Autodesk Fusion 360 part; units mm, degrees
(part 4 of 4)
sketch "Sketch10" plane through (0, 0, 4.8) normal (0, 0, 1) x (-1, 0, 0)
  circle A0 centre (0, 0) radius 3
  line L0 (57.7941, -61.1213) -> (57.7941, -86.8787)
  arc A1 (55.6728, -89) -> (57.7941, -86.8787) centre (56.7335, -87.9393) ccw
  line L1 (55.6728, -89) -> (53.2941, -89)
  line L2 (53.2941, -89) -> (53.2941, -89.8787)
  arc A2 (51.1728, -92) -> (53.2941, -89.8787) centre (52.2335, -90.9393) ccw
  line L3 (51.1728, -92) -> (18.4155, -92)
  arc A3 (16.2941, -89.8787) -> (18.4155, -92) centre (17.3548, -90.9393) ccw
  line L4 (16.2941, -89.8787) -> (16.2941, -89)
  line L5 (16.2941, -89) -> (13.9155, -89)
  arc A4 (11.7941, -86.8787) -> (13.9155, -89) centre (12.8548, -87.9393) ccw
  line L6 (11.7941, -86.8787) -> (11.7941, -61.1213)
  arc A5 (13.9155, -59) -> (11.7941, -61.1213) centre (12.8548, -60.0607) ccw
  line L7 (13.9155, -59) -> (16.2941, -59)
  line L8 (16.2941, -59) -> (16.2941, -58.1213)
  arc A6 (18.4155, -56) -> (16.2941, -58.1213) centre (17.3548, -57.0607) ccw
  line L9 (18.4155, -56) -> (51.1728, -56)
  arc A7 (53.2941, -58.1213) -> (51.1728, -56) centre (52.2335, -57.0607) ccw
  line L10 (53.2941, -58.1213) -> (53.2941, -59)
  line L11 (53.2941, -59) -> (55.6728, -59)
  arc A8 (57.7941, -61.1213) -> (55.6728, -59) centre (56.7335, -60.0607) ccw
  line L12 (51.1728, 56) -> (18.4155, 56)
  arc A9 (16.2941, 58.1213) -> (18.4155, 56) centre (17.3548, 57.0607) ccw
  line L13 (16.2941, 58.1213) -> (16.2941, 59)
  line L14 (16.2941, 59) -> (13.9155, 59)
  arc A10 (11.7941, 61.1213) -> (13.9155, 59) centre (12.8548, 60.0607) ccw
  line L15 (11.7941, 61.1213) -> (11.7941, 86.8787)
  arc A11 (13.9155, 89) -> (11.7941, 86.8787) centre (12.8548, 87.9393) ccw
  line L16 (13.9155, 89) -> (16.2941, 89)
  line L17 (16.2941, 89) -> (16.2941, 89.8787)
  arc A12 (18.4155, 92) -> (16.2941, 89.8787) centre (17.3548, 90.9393) ccw
  line L18 (18.4155, 92) -> (51.1728, 92)
  arc A13 (53.2941, 89.8787) -> (51.1728, 92) centre (52.2335, 90.9393) ccw
  line L19 (53.2941, 89.8787) -> (53.2941, 89)
  line L20 (53.2941, 89) -> (55.6728, 89)
  arc A14 (57.7941, 86.8787) -> (55.6728, 89) centre (56.7335, 87.9393) ccw
  line L21 (57.7941, 86.8787) -> (57.7941, 61.1213)
  arc A15 (55.6728, 59) -> (57.7941, 61.1213) centre (56.7335, 60.0607) ccw
  line L22 (55.6728, 59) -> (53.2941, 59)
  line L23 (53.2941, 59) -> (53.2941, 58.1213)
  arc A16 (51.1728, 56) -> (53.2941, 58.1213) centre (52.2335, 57.0607) ccw
  arc A17 (65.7941, 74.3) -> (67.2941, 72.8) centre (67.2941, 74.3) ccw
  line L24 (65.7941, 74.3) -> (65.7941, 100.26)
  arc A18 (68.1301, 101.5054) -> (65.7941, 100.26) centre (67.2941, 100.26) ccw
  arc A19 (96.3668, 75.223) -> (68.1301, 101.5054) centre (0, 0) ccw
  arc A20 (95.1844, 72.8) -> (96.3668, 75.223) centre (95.1844, 74.3) ccw
  line L25 (95.1844, 72.8) -> (67.2941, 72.8)
  arc A21 (65.7941, -100.26) -> (68.1301, -101.5054) centre (67.2941, -100.26) ccw
  line L26 (65.7941, -100.26) -> (65.7941, -74.3)
  arc A22 (67.2941, -72.8) -> (65.7941, -74.3) centre (67.2941, -74.3) ccw
  line L27 (67.2941, -72.8) -> (95.1844, -72.8)
  arc A23 (96.3668, -75.223) -> (95.1844, -72.8) centre (95.1844, -74.3) ccw
  arc A24 (68.1301, -101.5054) -> (96.3668, -75.223) centre (0, 0) ccw
  circle A25 centre (64.2941, -62.4) radius 1.5
  circle A26 centre (64.2941, 62.4) radius 1.5
  circle A27 centre (97.2941, -62.4) radius 1.5
  circle A28 centre (97.2941, 62.4) radius 1.5
  circle A29 centre (1.7941, -104.2) radius 6.1
  line L28 (15.4941, 111.4) -> (41.8941, 111.4)
  arc A30 (45.5941, 107.7) -> (41.8941, 111.4) centre (41.8941, 107.7) ccw
  line L29 (45.5941, 107.7) -> (45.5941, 100.7)
  arc A31 (41.8941, 97) -> (45.5941, 100.7) centre (41.8941, 100.7) ccw
  line L30 (41.8941, 97) -> (15.4941, 97)
  arc A32 (11.7941, 100.7) -> (15.4941, 97) centre (15.4941, 100.7) ccw
  line L31 (11.7941, 100.7) -> (11.7941, 107.7)
  arc A33 (15.4941, 111.4) -> (11.7941, 107.7) centre (15.4941, 107.7) ccw
  line L32 (15.4941, -97) -> (41.8941, -97)
  arc A34 (45.5941, -100.7) -> (41.8941, -97) centre (41.8941, -100.7) ccw
  line L33 (45.5941, -100.7) -> (45.5941, -107.7)
  arc A35 (41.8941, -111.4) -> (45.5941, -107.7) centre (41.8941, -107.7) ccw
  line L34 (41.8941, -111.4) -> (15.4941, -111.4)
  arc A36 (11.7941, -107.7) -> (15.4941, -111.4) centre (15.4941, -107.7) ccw
  line L35 (11.7941, -107.7) -> (11.7941, -100.7)
  arc A37 (15.4941, -97) -> (11.7941, -100.7) centre (15.4941, -100.7) ccw
  arc A38 (94.6728, -10) -> (96.7941, -7.8787) centre (95.7335, -8.9393) ccw
  line L36 (94.6728, -10) -> (94.1155, -10)
  arc A39 (91.9941, -7.8787) -> (94.1155, -10) centre (93.0548, -8.9393) ccw
  line L37 (91.9941, -7.8787) -> (91.9941, 7.8787)
  arc A40 (94.1155, 10) -> (91.9941, 7.8787) centre (93.0548, 8.9393) ccw
  line L38 (94.1155, 10) -> (94.6728, 10)
  arc A41 (96.7941, 7.8787) -> (94.6728, 10) centre (95.7335, 8.9393) ccw
  line L39 (96.7941, 7.8787) -> (96.7941, -7.8787)
  circle A42 centre (-94.9024, 87.3758) radius 1.5
  circle A43 centre (123.1209, -38.5) radius 1.5
  circle A44 centre (45.4941, 42.5) radius 1.5
  circle A45 centre (45.4941, -42.5) radius 1.5
  circle A46 centre (123.1209, 38.5) radius 1.5
  circle A47 centre (64.5, -111.7173) radius 1.5
  circle A48 centre (-28.2185, 125.8758) radius 1.5
  circle A49 centre (-94.9024, -87.3758) radius 1.5
  circle A50 centre (-28.2185, -125.8758) radius 1.5
  circle A51 centre (64.5, 111.7173) radius 1.5
  circle A52 centre (-123.5112, -37.2289) radius 1.5
  circle A53 centre (-123.5112, 37.2289) radius 1.5
  arc A54 (-55.2202, 79.8868) -> (-55.9967, 76.9891) centre (-55.6084, 78.438) ccw
  line L40 (-55.2202, 79.8868) -> (-41.5739, 87.7655)
  arc A55 (-38.6762, 86.9891) -> (-41.5739, 87.7655) centre (-40.125, 87.3773) ccw
  line L41 (-38.6762, 86.9891) -> (-38.3975, 86.5064)
  arc A56 (-39.1739, 83.6086) -> (-38.3975, 86.5064) centre (-38.7857, 85.0575) ccw
  line L42 (-39.1739, 83.6086) -> (-52.8202, 75.7299)
  arc A57 (-55.718, 76.5064) -> (-52.8202, 75.7299) centre (-54.2691, 76.1181) ccw
  line L43 (-55.718, 76.5064) -> (-55.9967, 76.9891)
  arc A58 (-11.2762, 39.5309) -> (-14.1739, 40.3073) centre (-12.725, 39.9191) ccw
  line L44 (-11.2762, 39.5309) -> (-10.9975, 39.0482)
  arc A59 (-11.7739, 36.1504) -> (-10.9975, 39.0482) centre (-11.3857, 37.5993) ccw
  line L45 (-11.7739, 36.1504) -> (-25.4202, 28.2717)
  arc A60 (-28.318, 29.0482) -> (-25.4202, 28.2717) centre (-26.8691, 28.66) ccw
  line L46 (-28.318, 29.0482) -> (-28.5967, 29.5309)
  arc A61 (-27.8202, 32.4286) -> (-28.5967, 29.5309) centre (-28.2084, 30.9798) ccw
  line L47 (-27.8202, 32.4286) -> (-14.1739, 40.3073)
  arc A62 (-10.9975, -39.0482) -> (-11.7739, -36.1504) centre (-11.3857, -37.5993) ccw
  line L48 (-10.9975, -39.0482) -> (-11.2762, -39.5309)
  arc A63 (-14.1739, -40.3073) -> (-11.2762, -39.5309) centre (-12.725, -39.9191) ccw
  line L49 (-14.1739, -40.3073) -> (-27.8202, -32.4286)
  arc A64 (-28.5967, -29.5309) -> (-27.8202, -32.4286) centre (-28.2084, -30.9798) ccw
  line L50 (-28.5967, -29.5309) -> (-28.318, -29.0482)
  arc A65 (-25.4202, -28.2717) -> (-28.318, -29.0482) centre (-26.8691, -28.66) ccw
  line L51 (-25.4202, -28.2717) -> (-11.7739, -36.1504)
  arc A66 (-52.8202, -75.7299) -> (-55.718, -76.5064) centre (-54.2691, -76.1181) ccw
  line L52 (-52.8202, -75.7299) -> (-39.1739, -83.6086)
  arc A67 (-38.3975, -86.5064) -> (-39.1739, -83.6086) centre (-38.7857, -85.0575) ccw
  line L53 (-38.3975, -86.5064) -> (-38.6762, -86.9891)
  arc A68 (-41.5739, -87.7655) -> (-38.6762, -86.9891) centre (-40.125, -87.3773) ccw
  line L54 (-41.5739, -87.7655) -> (-55.2202, -79.8868)
  arc A69 (-55.9967, -76.9891) -> (-55.2202, -79.8868) centre (-55.6084, -78.438) ccw
  line L55 (-55.9967, -76.9891) -> (-55.718, -76.5064)
  arc A70 (39.8728, -10) -> (41.9941, -7.8787) centre (40.9335, -8.9393) ccw
  line L56 (39.8728, -10) -> (39.3155, -10)
  arc A71 (37.1941, -7.8787) -> (39.3155, -10) centre (38.2548, -8.9393) ccw
  line L57 (37.1941, -7.8787) -> (37.1941, 7.8787)
  arc A72 (39.3155, 10) -> (37.1941, 7.8787) centre (38.2548, 8.9393) ccw
  line L58 (39.3155, 10) -> (39.8728, 10)
  arc A73 (41.9941, 7.8787) -> (39.8728, 10) centre (40.9335, 8.9393) ccw
  line L59 (41.9941, 7.8787) -> (41.9941, -7.8787)
  line L60 (-42.1213, -25.5) -> (-109.5263, -25.5)
  arc A74 (-109.5263, -25.5) -> (-110.7763, -25.8349) centre (-109.5263, -28) ccw
  line L61 (-110.7763, -25.8349) -> (-125.9451, -34.5927)
  arc A75 (-125.9451, -34.5927) -> (-127.0931, -37.4646) centre (-124.6951, -36.7577) ccw
  arc A76 (-127.0931, -37.4646) -> (-89.0244, -98.1371) centre (0, 0) ccw
  arc A77 (-89.0244, -98.1371) -> (-85.1797, -97.5355) centre (-87.3447, -96.2855) ccw
  line L62 (-85.1797, -97.5355) -> (-74.6084, -79.2255)
  arc A78 (-71.7106, -78.449) -> (-74.6084, -79.2255) centre (-73.1595, -78.8372) ccw
  line L63 (-71.7106, -78.449) -> (-32.0836, -101.3277)
  arc A79 (-31.3071, -104.2255) -> (-32.0836, -101.3277) centre (-31.6953, -102.7766) ccw
  line L64 (-31.3071, -104.2255) -> (-41.8784, -122.5355)
  arc A80 (-41.8784, -122.5355) -> (-40.477, -126.166) centre (-39.7133, -123.7855) ccw
  arc A81 (-40.477, -126.166) -> (129.5015, -28.0288) centre (0, 0) ccw
  arc A82 (129.5015, -28.0288) -> (127.0581, -25) centre (127.0581, -27.5) ccw
  line L65 (127.0581, -25) -> (105.9155, -25)
  arc A83 (103.7941, -22.8787) -> (105.9155, -25) centre (104.8548, -23.9393) ccw
  line L66 (103.7941, -22.8787) -> (103.7941, 22.8787)
  arc A84 (105.9155, 25) -> (103.7941, 22.8787) centre (104.8548, 23.9393) ccw
  line L67 (105.9155, 25) -> (127.0581, 25)
  arc A85 (127.0581, 25) -> (129.5015, 28.0288) centre (127.0581, 27.5) ccw
  arc A86 (129.5015, 28.0288) -> (-40.477, 126.166) centre (0, 0) ccw
  arc A87 (-40.477, 126.166) -> (-41.8784, 122.5355) centre (-39.7133, 123.7855) ccw
  line L68 (-41.8784, 122.5355) -> (-31.3071, 104.2255)
  arc A88 (-32.0836, 101.3277) -> (-31.3071, 104.2255) centre (-31.6953, 102.7766) ccw
  line L69 (-32.0836, 101.3277) -> (-71.7106, 78.449)
  arc A89 (-74.6084, 79.2255) -> (-71.7106, 78.449) centre (-73.1595, 78.8372) ccw
  line L70 (-74.6084, 79.2255) -> (-85.1797, 97.5355)
  arc A90 (-85.1797, 97.5355) -> (-89.0244, 98.1371) centre (-87.3447, 96.2855) ccw
  arc A91 (-89.0244, 98.1371) -> (-127.0931, 37.4646) centre (0, 0) ccw
  arc A92 (-127.0931, 37.4646) -> (-125.9451, 34.5927) centre (-124.6951, 36.7577) ccw
  line L71 (-125.9451, 34.5927) -> (-110.7763, 25.8349)
  arc A93 (-110.7763, 25.8349) -> (-109.5263, 25.5) centre (-109.5263, 28) ccw
  line L72 (-109.5263, 25.5) -> (-42.1213, 25.5)
  arc A94 (-40, 23.3787) -> (-42.1213, 25.5) centre (-41.0607, 24.4393) ccw
  line L73 (-40, 23.3787) -> (-40, 20.8)
  arc A95 (-40, 20.8) -> (-37.5, 18.3) centre (-37.5, 20.8) ccw
  line L74 (-37.5, 18.3) -> (-34.1213, 18.3)
  arc A96 (-32, 16.1787) -> (-34.1213, 18.3) centre (-33.0607, 17.2393) ccw
  line L75 (-32, 16.1787) -> (-32, -16.1787)
  arc A97 (-34.1213, -18.3) -> (-32, -16.1787) centre (-33.0607, -17.2393) ccw
  line L76 (-34.1213, -18.3) -> (-37.5, -18.3)
  arc A98 (-37.5, -18.3) -> (-40, -20.8) centre (-37.5, -20.8) ccw
  line L77 (-40, -20.8) -> (-40, -23.3787)
  arc A99 (-42.1213, -25.5) -> (-40, -23.3787) centre (-41.0607, -24.4393) ccw
  line L78 (-42.1213, 25.5) -> (-109.5263, 25.5)
  line L79 (-42.1213, -25.5) -> (-109.5263, -25.5)
  arc A100 (-127.0931, -37.4646) -> (-89.0244, -98.1371) centre (0, 0) ccw
  arc A101 (-89.0244, 98.1371) -> (-127.0931, 37.4646) centre (0, 0) ccw
  line L80 (-25.6319, 7.5958) -> (-67.8319, 80.6884)
  line L81 (-25.6319, -7.5958) -> (-67.8319, -80.6884)
  circle A102 centre (-53.2894, 35.5) radius 1.5
  circle A103 centre (-100, 35.5) radius 1.5
  line L82 (-130.0231, 25.5) -> (-40, 25.5)
  line L83 (-100, 25.5) -> (-100, -25.5) construction
  line L84 (-40, 25.5) -> (-40, -25.5) construction
  line L85 (-100, 25.5) -> (-100, 35.5) construction
  circle A104 centre (-53.2894, -35.5) radius 1.5
  circle A105 centre (-100, -35.5) radius 1.5
  line L86 (-100, -25.5) -> (-100, -35.5) construction
  line L87 (-103, 28.5) -> (-103, 35.5)
  line L88 (-100, 38.5) -> (-48.1666, 38.5)
  line L89 (0, 0) -> (-44.1633, 38.5) construction
  line L90 (-47.1809, 41.1307) -> (-97.2023, 84.7376)
  line L91 (-85.1797, 97.5355) -> (-74.6084, 79.2255)
  line L92 (-103, 25.5) -> (-103, 28.5) construction
  arc A106 (-100, 25.5) -> (-103, 28.5) centre (-100, 28.5) ccw construction
  arc A107 (-103, 28.5) -> (-100, 25.5) centre (-100, 28.5) ccw
  arc A108 (-48.1666, 38.5) -> (-47.1809, 41.1307) centre (-48.1666, 40) ccw
  arc A109 (-100, 38.5) -> (-103, 35.5) centre (-100, 35.5) ccw
  arc A110 (-40.477, 126.166) -> (-40.477, -126.166) centre (0, 0) ccw
  line L93 (-97.2023, 84.7376) -> (-99.8764, 87.0687) construction
  arc A111 (-97.2023, 84.7376) -> (-97.4773, 89.7465) centre (-94.9024, 87.3758) ccw construction
  arc A112 (-97.4773, 89.7465) -> (-97.2023, 84.7376) centre (-94.9024, 87.3758) ccw
  line L94 (0, 0) -> (-44.1633, -38.5) construction
  line L95 (-48.1666, -38.5) -> (-100, -38.5)
  line L96 (-103, -35.5) -> (-103, -28.5)
  line L97 (-47.1809, -41.1307) -> (-97.2023, -84.7376)
  arc A113 (-47.1809, -41.1307) -> (-48.1666, -38.5) centre (-48.1666, -40) ccw
  arc A114 (-103, -35.5) -> (-100, -38.5) centre (-100, -35.5) ccw
  arc A115 (-97.4773, -89.7465) -> (-97.2023, -84.7376) centre (-94.9024, -87.3758) ccw construction
  arc A116 (-97.2023, -84.7376) -> (-97.4773, -89.7465) centre (-94.9024, -87.3758) ccw
  line L98 (-97.2023, -84.7376) -> (-99.8764, -87.0687) construction
  line L99 (-40, -25.5) -> (-130.0231, -25.5)
  arc A117 (-100, -31.5) -> (-100, -25.5) centre (-100, -28.5) ccw construction
  arc A118 (-100, -25.5) -> (-103, -28.5) centre (-100, -28.5) ccw
  arc A119 (-103, -28.5) -> (-100, -31.5) centre (-100, -28.5) ccw construction
  line L100 (-103, -28.5) -> (-103, -25.5) construction
  point P0 (-94.9024, 87.3758)
  point P1 (-94.9024, -87.3758)
  dimension "d371" = 3
  dimension "d372" = 3
  dimension "d373" = 10
  dimension "d374" = 10
  dimension "d375" = 10
  dimension "d376" = 60
  dimension "d377" = 3
  dimension "d378" = 3
  dimension "d379" = 10
  dimension "d380" = 10
  dimension "d381" = 10
  dimension "d383" = 3
  dimension "d384" = 3
  dimension "d385" = 6
  dimension "d386" = 1.5
  dimension "d387" = 3
  dimension "d388" = 7
  dimension "d389" = 3.5
  dimension "d390" = 3
  dimension "d391" = 3
  dimension "d392" = 3.5
  dimension "d393" = 1.5
  dimension "d394" = 3
  dimension "d395" = 3
  constraint coincident L82 L83.start
  constraint coincident L79 L83.end
  constraint perpendicular L79 L83
  constraint coincident A103.centre L85.end
  constraint vertical L85
  constraint coincident A105.centre L86.end
  constraint vertical L86
  constraint coincident L82 L92.start
  constraint perpendicular L82 L87
  constraint perpendicular L85 L88
  constraint coincident A0.centre A19.centre
  constraint coincident A101 L93.end
  constraint parallel L89 L90
  constraint tangent L87 A106
  constraint tangent L82 A106
  constraint perpendicular L82 L92
  constraint coincident L72 L83.start
  constraint concentric A106 A107
  constraint coincident L89.end L90
  constraint coincident L89.end L88
  constraint tangent L90 A108
  constraint tangent L88 A108
  constraint tangent L88 A109
  constraint tangent L87 A109
  constraint tangent L90 A111
  constraint tangent A110 A111
  constraint parallel L89 L93
  constraint coincident A91 A111.end
  constraint concentric A111 A112
  constraint coincident A100 L98.end
  constraint horizontal L95
  constraint coincident L79 L100.end
  constraint perpendicular L79 L96
  constraint coincident L94.end L97
  constraint coincident L94.end L95
  constraint tangent L97 A113
  constraint tangent L95 A113
  constraint tangent L95 A114
  constraint tangent L96 A114
  constraint coincident P1 A49.centre
  constraint tangent L97 A115
  constraint coincident A76 A115.start
  constraint concentric A115 A116
  constraint coincident L94.end L98
  constraint tangent L96 A117
  constraint tangent L99 A117
  constraint coincident L60 L83.end
  constraint concentric A117 A118
  constraint coincident L86 A117.start
  constraint concentric A117 A119
  constraint perpendicular L79 L100
  measures "d371" diameter of A102
  measures "d372" diameter of A103
  measures "d373" distance of L80 A102.centre
  measures "d374" distance of A102.centre L82
  measures "d375" distance of L78 A103.centre
  measures "d376" distance of L83 L84
  measures "d377" diameter of A104
  measures "d378" diameter of A105
  measures "d379" distance of L79 A105.centre
  measures "d380" distance of L79 A104.centre
  measures "d381" distance of L81 A104.centre
  measures "d383" distance of A103.centre L88
  measures "d384" distance of A103.centre L87
  measures "d385" diameter of A106
  measures "d386" radius of A108
  measures "d387" radius of A109
  measures "d388" diameter of A111
  measures "d389" distance of L90 P0
  measures "d390" distance of A105.centre L96
  measures "d391" distance of A105.centre L95
  measures "d392" distance of L94 P1
  measures "d393" radius of A113
  measures "d394" radius of A114
  measures "d395" radius of A118
extrude "Extrude13" cut sketch "Sketch10" against normal through all contours L60 A74 L61 A75 A76 L79 A100 A110 L95 L96 L97 A113 A114 A116 L99 A118 | A91 A92 L71 A93 L72 L78 A101 L82 L87 L88 L90 A107 A108 A109 A110 A112 | A102 | A103 | A104 | A105
